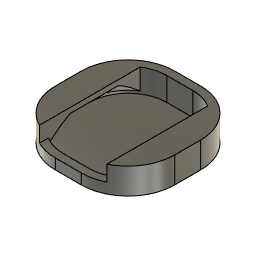
separator-point (Autodesk Fusion 360 design; units mm, degrees)
Autodesk Fusion 360 part; units mm, degrees
sketch "Esquisse1" plane through (0, 0, 0) normal (0, 0, 1) x (1, 0, 0)
  line L0 (7.5, 0) -> (12.5, 0)
  line L1 (20, 7.5) -> (20, 12.5)
  line L2 (12.5, 20) -> (7.5, 20)
  line L3 (0, 12.5) -> (0, 7.5)
  arc A0 (7.5, 20) -> (0, 12.5) centre (7.5, 12.5) ccw
  arc A1 (0, 7.5) -> (7.5, 0) centre (7.5, 7.5) ccw
  arc A2 (12.5, 0) -> (20, 7.5) centre (12.5, 7.5) ccw
  arc A3 (20, 12.5) -> (12.5, 20) centre (12.5, 12.5) ccw
  arc A4 (-1.5, 7.5) -> (7.5, -1.5) centre (7.5, 7.5) ccw
  line L4 (7.5, -1.5) -> (12.5, -1.5)
  arc A5 (12.5, -1.5) -> (21.5, 7.5) centre (12.5, 7.5) ccw
  line L5 (21.5, 7.5) -> (21.5, 12.5)
  arc A6 (21.5, 12.5) -> (12.5, 21.5) centre (12.5, 12.5) ccw
  line L6 (12.5, 21.5) -> (7.5, 21.5)
  arc A7 (7.5, 21.5) -> (-1.5, 12.5) centre (7.5, 12.5) ccw
  line L7 (-1.5, 12.5) -> (-1.5, 7.5)
  line L8 (3.5, 20) -> (16.5, 20)
  line L9 (16.5, 20) -> (16.5, -5)
  line L10 (16.5, -5) -> (3.5, -5)
  line L11 (3.5, -5) -> (3.5, 20)
  point P0 (20, 0)
  point P1 (0, 20)
  point P2 (10, 20)
  point P3 (10, 20)
  dimension "d1" = 20
  dimension "d2" = 20
  dimension "d3" = 7.5
  dimension "d4" = 1.5
  dimension "d5" = 13
  dimension "d6" = 25
  constraint horizontal L0
  constraint vertical L1
  constraint horizontal L2
  constraint vertical L3
  constraint coincident P1 L2
  constraint coincident P1 L3
  constraint tangent L2 A0
  constraint tangent L3 A0
  constraint coincident origin L3
  constraint coincident origin L0
  constraint tangent L3 A1
  constraint tangent L0 A1
  constraint equal A0 A1
  constraint coincident P0 L0
  constraint coincident P0 L1
  constraint tangent L0 A2
  constraint tangent L1 A2
  constraint equal A0 A2
  constraint tangent L2 A3
  constraint tangent L1 A3
  constraint equal A0 A3
  constraint horizontal L8
  constraint vertical L9
  constraint horizontal L10
  constraint vertical L11
  constraint collinear L2 L8
  constraint midpoint L2 P3
  constraint midpoint L8 P3
  constraint coincident P3 P2
  measures "d1" distance of origin P0
  measures "d2" distance of origin P1
  measures "d3" radius of A0
  measures "d5" distance of L8.start L8.end
  measures "d6" distance of L8.start L10.end
extrude "Extrusion1" add sketch "Esquisse1" along normal blind 5 contours L0 A1 A2 A4 L4 A5 L9 L11 | L1 L2 L3 A0 A1 A2 A3 A4 A5 L5 A6 L6 A7 L7 L8 L9 L11 | A0 L8 L11 | A3 L8 L9
extrude "Extrusion2" add sketch "Esquisse1" along normal blind 0.5 contours L0 L2 A0 A1 A2 A3 L8 L9 L11 | L3 A0 A1 L11 | L1 A2 A3 L9
extrude "Extrusion5" add sketch "Esquisse1" against normal blind 1 from surface at 5 contours L3 A0 A1 L11 | L1 A2 A3 L9
extrude "Extrusion3" cut sketch "Esquisse1" against normal blind 3 from surface at 5 contours L0 A1 A2 A4 L4 A5 L9 L11
sketch "Esquisse2" plane through (3.5, 0, 0) normal (1, 0, 0) x (0, 1, 0)
  line L0 (18.8443, 5) -> (-0.5623, 5)
  line L1 (-0.5623, 5) -> (-0.5623, 2)
  line L2 (-0.5623, 2) -> (1.1557, 2)
  line L3 (1.1557, 2) -> (1.1557, 4)
  line L4 (17.8443, 4) -> (1.8443, 4)
  line L5 (1.8443, 4) -> (1.8443, 1)
  line L6 (1.8443, 1) -> (17.8443, 1)
  line L7 (17.8443, 1) -> (17.8443, 4)
  line L8 (1.1557, 4) -> (18.8443, 4)
  line L9 (18.8443, 4) -> (18.8443, 5)
  dimension "d15" = 1
  dimension "d16" = 16
  dimension "d17" = 3
  constraint horizontal L4
  constraint vertical L5
  constraint horizontal L6
  constraint vertical L7
  measures "d15" distance of L0 L4
  measures "d16" distance of L4.start L4.end
  measures "d17" distance of L4 L6
extrude "Extrusion4" cut sketch "Esquisse2" along normal blind -0.5 and the other way blind -13.5 contours L4 L5 L6 L7 L8
chamfer "Chanfrein1" distance 3 angle 45 3 edges at (0, 10, 4) (0.933, 3.8772, 4) (0.933, 16.1228, 4)
chamfer "Chanfrein1" distance 3 angle 45 3 edges at (20, 10, 4) (19.067, 16.1228, 4) (19.067, 3.8772, 4)
